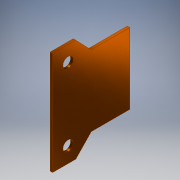
# Autodesk Inventor part: Для иконки
Saved by Autodesk Inventor 2018.2 (Build 222227000, 227)
## iProperties
Created: 2020-04-26
Part Number: Для иконки
Material: Медь
Document SubType Name: Modeling
Designer: 79992
Density: 8.94 g/cm^3
Appearance: Лощеная
Mass: 67.9345 g
Surface Area: 82.3078 cm^2
Volume: 7.59894 cm^3
Author: 79992
Autodesk Inventor part; units mm, degrees
ref_plane "YZ Plane" through (0, 0, 0) normal (1, 0, 0) x (0, 1, 0)
ref_plane "XZ Plane" through (0, 0, 0) normal (0, 1, 0) x (-1, 0, 0)
ref_plane "XY Plane" through (0, 0, 0) normal (0, 0, 1) x (1, 0, 0)
sketch "Эскиз1" plane through (0, 0, 0) normal (1, 0, 0) x (0, 1, 0)
  line L0 (-30, 0) -> (30, 0)
  line L1 (-30, 0) -> (-30, 40)
  line L2 (-30, 40) -> (-12, 40)
  line L3 (30, 0) -> (30, 27.5)
  line L4 (30, 27.5) -> (0, 27.5)
  line L5 (0, 27.5) -> (-12, 40)
  circle A0 centre (-18, 28) radius 4
  line L6 (-30, 0) -> (-30, -40)
  line L7 (-30, -40) -> (-12, -40)
  line L8 (30, 0) -> (30, -27.5)
  line L9 (30, -27.5) -> (0, -27.5)
  line L10 (0, -27.5) -> (-12, -40)
  circle A1 centre (-18, -28) radius 4
  point P0 (0, 0)
  point P1 (0, 0)
  dimension "d1" = 40
  dimension "d2" = 18
  dimension "d3" = 55
  dimension "d4" = 30
  dimension "d5" = 60
  dimension "d6" = 8
  dimension "d7" = 12
  dimension "d8" = 12
  constraints: 22 end point, 5 symmetric about line, 2 centre point, 2 horizontal, 2 vertical, 1 coincident, 1 midpoint, 1 perpendicular, 1 other
  measures "d1" distance of L0.start L1.end
  measures "d2" distance of L1.end L2.end
  measures "d3" diameter of L3.end L0
  measures "d4" distance of L3.end L4.end
  measures "d5" distance between parallel lines of L1 L3
  measures "d6" diameter of A0
  measures "d7" distance from line of L2 A0.centre
  measures "d8" distance from line of L1 A0.centre
extrude "Выдавливание1" add sketch "Эскиз1" along normal blind 2
